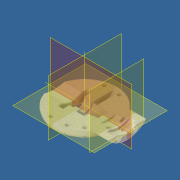
# Autodesk Inventor part: Wrist_B_r1
Saved by Autodesk Inventor 2016 (Build 200138000, 138)
## iProperties
Created: 2016-03-10
Part Number: Wrist_B_r1
Material: ABS-Kunststoff
Document SubType Name: Modeling
Designer: 4ndreas
Density: 1.06 g/cm^3
Appearance: Glatt - weiß
Author: 4ndreas
Autodesk Inventor part; units mm, degrees
sketch "Skizze1" plane through (0, 0, 0) normal (0, 0, 1) x (1, 0, 0)
  circle A0 centre (0, 0) radius 37.5
  line L0 (0, 0) -> (0, 37.5) construction
  dimension "d0" = 75
  constraints: 2 end point, 1 coincident, 1 vertical, 1 vertical alignment, 2 other
extrude "Extrusion1" add sketch "Skizze1" along normal mid plane 58
ref_plane "Arbeitsebene1" through (0, 0, 0) normal (1, 0, 0) x (0, 1, 0)
sketch "Skizze2" plane through (0, 0, 0) normal (1, 0, 0) x (0, 1, 0)
  line L0 (37.5, -29) -> (-37.5, -29) projected
  line L1 (-37.5, -29) -> (-37.5, 29) projected
  line L2 (-37.5, 29) -> (37.5, 29) projected
  line L3 (37.5, 29) -> (37.5, -29) projected
  circle A0 centre (0, 0) radius 29
  constraints: 1 centre point, 1 coincident, 1 tangent
extrude "Extrusion2" add sketch "Skizze2" along normal blind 50 contours A0
ref_plane "Arbeitsebene2" through (0, 0, 0) normal (0, 0, -1) x (-1, 0, 0)
sketch "Skizze3" plane through (50, 0, 0) normal (1, 0, 0) x (0, 0, -1)
  circle A0 centre (0, 0) radius 23.5
  dimension "d7" = 47
  constraints: 1 centre point, 1 coincident
  measures "d7" diameter of A0
extrude "Extrusion3" cut sketch "Skizze3" against normal blind 10
sketch "Skizze4" plane through (40, 0, 0) normal (1, 0, 0) x (0, 0, -1)
  circle A0 centre (0, 0) radius 21
  point P0 (0, 0)
  dimension "d10" = 42
  constraints: 1 centre point, 1 coincident
  measures "d10" diameter of A0
extrude "Extrusion4" cut sketch "Skizze4" against normal blind 12
ref_plane "Arbeitsebene3" through (0, 0, 0) normal (0, -1, 0) x (1, 0, 0)
sketch "Skizze5" plane through (50, 0, 0) normal (1, 0, 0) x (0, 0, -1)
  point P0 (0, 0)
ref_plane "Arbeitsebene4" through (0, 0, 0) normal (1, 0, 0) x (0, 1, 0)
sketch "Skizze6" plane through (0, 0, 0) normal (1, 0, 0) x (0, 1, 0)
  circle A0 centre (20.5107, -9.25) radius 3
  circle A1 centre (0, -18.5) radius 3
  point P0 (0, 0)
  dimension "d13" = 6
  constraints: 2 centre point, 2 coincident, 1 equal radius, 2 other
  measures "d13" diameter of A0
extrude "Extrusion5" cut sketch "Skizze6" along normal mid plane 30
ref_plane "Arbeitsebene5" through (-35, 0, 0) normal (-1, 0, 0) x (0, 1, 0)
ref_plane "Arbeitsebene6" through (-15, 0, 0) normal (1, 0, 0) x (0, -1, 0)
sketch "Skizze8" plane through (-15, 0, 0) normal (1, 0, 0) x (0, -1, 0)
  circle A0 centre (0, 0) radius 5 projected
  circle A1 centre (-25, 0) radius 1.75 projected
  line L0 (14.49, -15.2) -> (27.5875, -2.7143) projected
  arc A2 (27.5875, -2.7143) -> (27.5875, 2.7143) centre (25, 0) ccw projected
  line L1 (27.5875, 2.7143) -> (14.49, 15.2) projected
  arc A3 (14.49, 15.2) -> (-14.49, 15.2) centre (0, 0) ccw projected
  line L2 (-14.49, 15.2) -> (-27.5875, 2.7143) projected
  arc A4 (-27.5875, 2.7143) -> (-27.5875, -2.7143) centre (-25, 0) ccw projected
  line L3 (-27.5875, -2.7143) -> (-14.49, -15.2) projected
  arc A5 (-14.49, -15.2) -> (14.49, -15.2) centre (0, 0) ccw projected
  circle A6 centre (25, 0) radius 1.75 projected
  point P0 (0, 0)
extrude "Extrusion6" cut sketch "Skizze8" against normal through all contours A0 | A1 | A5 L3 A4 L2 A3 L1 A2 L0 | A6
sketch "Skizze9" plane through (28, 0, 0) normal (1, 0, 0) x (0, 0, -1)
  circle A0 centre (0, 0) radius 11
  point P0 (0, 0)
  dimension "d18" = 22
  constraints: 1 centre point, 1 coincident
  measures "d18" diameter of A0
extrude "Extrusion7" cut sketch "Skizze9" against normal blind 7
sketch "Skizze10" plane through (21, 0, 0) normal (1, 0, 0) x (0, 0, -1)
  circle A0 centre (0, 0) radius 6.5
  point P0 (0, 0)
  dimension "d21" = 13
  constraints: 1 centre point, 1 coincident
  measures "d21" diameter of A0
extrude "Extrusion8" cut sketch "Skizze10" against normal through all
ref_plane "Arbeitsebene7" through (50, 0, 0) normal (0, 1, 0) x (-1, 0, 0)
sketch "Skizze11" plane through (50, 0, 0) normal (0, 1, 0) x (-1, 0, 0)
  line L0 (87.5, -29) -> (12.5, -29) projected
  line L1 (0, -29) -> (0, -23.5) projected
  line L2 (0, -23.5) -> (10, -23.5) projected
  line L3 (10, -23.5) -> (10, -21) projected
  line L4 (10, -21) -> (22, -21) projected
  line L5 (22, -21) -> (22, -11) projected
  line L6 (22, -11) -> (29, -11) projected
  line L7 (29, -11) -> (29, -6.5) projected
  line L8 (29, -6.5) -> (65, -6.5) projected
  line L9 (65, 6.5) -> (29, 6.5) projected
  line L10 (29, 6.5) -> (29, 11) projected
  line L11 (29, 11) -> (22, 11) projected
  line L12 (22, 11) -> (22, 21) projected
  line L13 (22, 21) -> (10, 21) projected
  line L14 (10, 21) -> (10, 23.5) projected
  line L15 (10, 23.5) -> (0, 23.5) projected
  line L16 (0, 23.5) -> (0, 29) projected
  line L17 (12.5, 29) -> (87.5, 29) projected
  line L18 (87.5, 29) -> (87.5, 21) projected
  line L19 (87.5, 21) -> (65, 21) projected
  line L20 (65, 21) -> (65, 6.5) projected
  line L21 (65, -15.5) -> (35, -15.5) projected
  line L22 (35, -15.5) -> (35, -21.5) projected
  line L23 (35, -21.5) -> (65, -21.5) projected
  line L24 (65, -21.5) -> (65, -21) projected
  line L25 (65, -21) -> (87.5, -21) projected
  line L26 (87.5, -21) -> (87.5, -29) projected
  line L27 (31, 0) -> (29, 0)
  line L28 (29, 0) -> (29, 9.5)
  line L29 (29, 9.5) -> (31, 9.5)
  line L30 (31, 9.5) -> (31, 0)
  line L31 (87.5, -29) -> (12.5, -29) projected
  line L32 (12.5, -29) -> (0, -29) projected
  line L33 (0, -29) -> (0, -23.5) projected
  line L34 (0, -23.5) -> (10, -23.5) projected
  line L35 (29, -6.5) -> (65, -6.5) projected
  line L36 (65, 6.5) -> (29, 6.5) projected
  line L37 (10, 23.5) -> (0, 23.5) projected
  line L38 (0, 23.5) -> (0, 29) projected
  line L39 (0, 29) -> (12.5, 29) projected
  line L40 (12.5, 29) -> (87.5, 29) projected
  line L41 (87.5, 29) -> (87.5, 21) projected
  line L42 (87.5, 21) -> (65, 21) projected
  line L43 (65, 21) -> (65, 6.5) projected
  line L44 (65, -15.5) -> (35, -15.5) projected
  line L45 (65, -21) -> (87.5, -21) projected
  line L46 (87.5, -21) -> (87.5, -29) projected
  line L47 (-17.7485, 0) -> (106.4912, 0) projected
  line L48 (65, -6.5) -> (65, -15.5) projected
  line L49 (65, -6.5) -> (65, -15.5) projected
  line L50 (35, -15.5) -> (35, -21.5) projected
  line L51 (35, -21.5) -> (65, -21.5) projected
  line L52 (65, -21.5) -> (65, -21) projected
  line L53 (29, 6.5) -> (29, 11) projected
  line L54 (29, 11) -> (22, 11) projected
  line L55 (22, 11) -> (22, 21) projected
  line L56 (22, 21) -> (10, 21) projected
  line L57 (10, 21) -> (10, 23.5) projected
  line L58 (10, -23.5) -> (10, -21) projected
  line L59 (10, -21) -> (22, -21) projected
  line L60 (22, -21) -> (22, -11) projected
  line L61 (22, -11) -> (29, -11) projected
  line L62 (29, -11) -> (29, -6.5) projected
  line L63 (12.5, -29) -> (0, -29) projected
  line L64 (0, 29) -> (12.5, 29) projected
  point P0 (50, 0)
  dimension "d25" = 2
  dimension "d66" = 19
  constraints: 8 end point, 2 collinear, 2 parallel, 1 horizontal, 1 perpendicular
  measures "d25" distance between parallel lines of L30 L28
  measures "d66" diameter of L29 L47
revolve "Umdrehung1" cut sketch "Skizze11" angle 360 about axis through (50, 0, 0) along (-1, 0, 0) contours L30 L27 L28 L9 | L9 L10 L29 L30
ref_plane "Arbeitsebene8" through (50, 0, 0) normal (0, 0, -1) x (-1, 0, 0)
ref_plane "Arbeitsebene9" through (0, 20.5107, -9.25) normal (0, -0.4111111, -0.9115852) x (1, 0, 0)
sketch "Skizze12" plane through (50, 0, 0) normal (0, 1, 0) x (-1, 0, 0)
  line L0 (87.5, 29) -> (87.5, 21) projected
  line L1 (87.5, 21) -> (65, 21) projected
  line L2 (65, 21) -> (65, 6.5) projected
  line L3 (65, 6.5) -> (31, 6.5) projected
  line L4 (31, 6.5) -> (31, 9.5) projected
  line L5 (31, 9.5) -> (29, 9.5) projected
  line L6 (29, 9.5) -> (29, 11) projected
  line L7 (29, 11) -> (22, 11) projected
  line L8 (22, 11) -> (22, 21) projected
  line L9 (22, 21) -> (10, 21) projected
  line L10 (10, 21) -> (10, 23.5) projected
  line L11 (10, 23.5) -> (0, 23.5) projected
  line L12 (0, 23.5) -> (0, 29) projected
  line L13 (12.5, 29) -> (87.5, 29) projected
  line L14 (87.5, -29) -> (12.5, -29) projected
  line L15 (0, -29) -> (0, -23.5) projected
  line L16 (0, -23.5) -> (10, -23.5) projected
  line L17 (10, -23.5) -> (10, -21) projected
  line L18 (10, -21) -> (22, -21) projected
  line L19 (22, -21) -> (22, -11) projected
  line L20 (22, -11) -> (29, -11) projected
  line L21 (29, -11) -> (29, -9.5) projected
  line L22 (29, -9.5) -> (31, -9.5) projected
  line L23 (31, -9.5) -> (31, -6.5) projected
  line L24 (31, -6.5) -> (65, -6.5) projected
  line L25 (65, -6.5) -> (65, -15.5) projected
  line L26 (65, -15.5) -> (35, -15.5) projected
  line L27 (35, -15.5) -> (35, -21.5) projected
  line L28 (35, -21.5) -> (65, -21.5) projected
  line L29 (65, -21.5) -> (65, -21) projected
  line L30 (65, -21) -> (87.5, -21) projected
  line L31 (87.5, -21) -> (87.5, -29) projected
  line L32 (105, -18.5) -> (-17.5, -18.5) projected
  line L33 (54, -18.5) -> (34, -18.5)
  line L34 (34, -18.5) -> (34, -25)
  line L35 (34, -25) -> (54, -25)
  line L36 (54, -25) -> (54, -18.5)
  line L37 (65, -20.9257) -> (65, -15.5) projected
  line L38 (49, -25) -> (39, -25)
  line L39 (39, -25) -> (39, -27.5)
  line L40 (39, -27.5) -> (49, -27.5)
  line L41 (49, -27.5) -> (49, -25)
  line L42 (54, -27.5) -> (59, -27.5)
  line L43 (59, -27.5) -> (59, -18.5)
  line L44 (59, -18.5) -> (54, -18.5)
  line L45 (54, -18.5) -> (54, -27.5)
  line L46 (59, -18.5) -> (65, -18.5)
  line L47 (65, -18.5) -> (65, -35)
  line L48 (65, -35) -> (59, -35)
  line L49 (59, -35) -> (59, -18.5)
  line L50 (12.5, -29) -> (0, -29) projected
  line L51 (0, 29) -> (12.5, 29) projected
  line L52 (54, -27.5) -> (59, -27.5)
  line L53 (59, -27.5) -> (59, -18.5)
  line L54 (59, -18.5) -> (54, -18.5)
  line L55 (54, -18.5) -> (54, -27.5)
  line L56 (34, -18.5) -> (39, -18.5)
  line L57 (39, -18.5) -> (39, -25)
  line L58 (39, -25) -> (34, -25)
  line L59 (34, -25) -> (34, -18.5)
  line L60 (34, -18.5) -> (29, -18.5)
  line L61 (29, -18.5) -> (29, -24)
  line L62 (29, -24) -> (34, -24)
  line L63 (34, -24) -> (34, -18.5)
  line L64 (54, -18.5) -> (48, -18.5)
  line L65 (48, -18.5) -> (48, -28)
  line L66 (48, -28) -> (54, -28)
  line L67 (54, -28) -> (54, -18.5)
  point P0 (50, 0)
  dimension "d30" = 20
  dimension "d31" = 11
  dimension "d57" = 5
  dimension "d58" = 5
  dimension "d59" = 18
  dimension "d60" = 33
  dimension "d61" = 5
  dimension "d62" = 6
  dimension "d136" = 13
  dimension "d142" = 13
  dimension "d143" = 5
  dimension "d144" = 18
  dimension "d145" = 11
  dimension "d146" = 19
  dimension "d147" = 6
  constraints: 64 end point, 16 parallel, 8 horizontal, 8 perpendicular, 5 point on line, 2 collinear
  measures "d30" distance between parallel lines of L34 L36
  measures "d31" distance between parallel lines of L36 L37
  measures "d57" distance between parallel lines of L36 L41
  measures "d58" distance between parallel lines of L39 L34
  measures "d59" diameter of L42 L32
  measures "d60" diameter of L48 L32
  measures "d61" distance between parallel lines of L43 L45
  measures "d62" distance between parallel lines of L47 L49
  measures "d136" diameter of L35 L32
  measures "d142" diameter of L58 L32
  measures "d143" distance between parallel lines of L34 L61
  measures "d144" diameter of L40 L32
  measures "d145" diameter of L62 L32
  measures "d146" diameter of L66 L32
  measures "d147" distance between parallel lines of L36 L65
revolve "Umdrehung2" cut sketch "Skizze12" angle 360 about axis through (0, 0, -18.5) along (1, 0, 0) contours L47 L48 L49 L14 | L14 L49 L43 L28 L47 | L28 L43 L32 L37 L47 L29 | L42 L45 L36 L28 L43 | L28 L36 L32 L43 | L36 L35 L65 L28 | L28 L65 L32 L36 | L65 L35 L57 L28 | L28 L57 L32 L65 | L41 L40 L65 L35 | L57 L35 L34 L32 L27 L28 | L28 L27 L32 L57 | L65 L40 L39 L35 | L34 L62 L61 L32
sketch "Skizze13" plane through (0, 20.5107, -9.25) normal (0, -0.4111111, -0.9115852) x (1, 0, 0)
  line L0 (-15, -1.2682) -> (-15, 0.9858) projected
  line L1 (-15, 0.9858) -> (-15, -1.2682) projected
  line L2 (15, -3) -> (15, 3) projected
  line L3 (-31.2952, -0.1645) -> (-15, -0.1645) projected
  line L4 (-15, -0.1645) -> (-15, -3) projected
  line L5 (-15, -3) -> (15, -3) projected
  line L6 (15, 3) -> (-15, 3) projected
  line L7 (-15, 3) -> (-15, 16) projected
  line L8 (-15, 16) -> (19, 16) projected
  line L9 (19, 16) -> (19, 13) projected
  line L10 (19, 13) -> (21, 13) projected
  line L11 (21, 13) -> (21, 11.5) projected
  line L12 (21, 11.5) -> (28, 11.5) projected
  line L13 (28, 11.5) -> (28, 1.5) projected
  line L14 (28, 1.5) -> (40, 1.5) projected
  line L15 (40, 1.5) -> (40, -1) projected
  line L16 (40, -1) -> (50, -1) projected
  line L17 (50, -1) -> (50, -6.5) projected
  line L18 (50, -6.5) -> (26.5968, -6.5) projected
  line L19 (26.5968, 51.5) -> (50, 51.5) projected
  line L20 (50, 51.5) -> (50, 46) projected
  line L21 (50, 46) -> (40, 46) projected
  line L22 (40, 46) -> (40, 43.5) projected
  line L23 (40, 43.5) -> (28, 43.5) projected
  line L24 (28, 43.5) -> (28, 33.5) projected
  line L25 (28, 33.5) -> (21, 33.5) projected
  line L26 (21, 33.5) -> (21, 32) projected
  line L27 (21, 32) -> (19, 32) projected
  line L28 (19, 32) -> (19, 29) projected
  line L29 (19, 29) -> (-15, 29) projected
  line L30 (-15, 29) -> (-15, 45.1645) projected
  line L31 (-15, 45.1645) -> (-31.2952, 45.1645) projected
  line L32 (-55, 0) -> (67.5, 0) projected
  line L33 (24, 0) -> (-4, 0)
  line L34 (-4, 0) -> (-4, 6.5)
  line L35 (-4, 6.5) -> (14, 6.5)
  line L36 (24, 6.5) -> (24, 0)
  line L37 (-15, 3) -> (-15, -1.2682) projected
  line L38 (28, 0) -> (24, 0)
  line L39 (24, 0) -> (24, 8)
  line L40 (24, 8) -> (28, 8)
  line L41 (28, 8) -> (28, 0)
  line L42 (34, 0) -> (28, 0)
  line L43 (28, 0) -> (28, 9)
  line L44 (28, 9) -> (34, 9)
  line L45 (34, 9) -> (34, 0)
  line L46 (1, 0) -> (7, 0)
  line L47 (7, 0) -> (7, 16)
  line L48 (7, 16) -> (1, 16)
  line L49 (1, 16) -> (1, 0)
  ellipse E0 centre (0, 22.5) end of major axis (0, 63.6371) minor radius 37.5 (-31.2952, -0.1645) -> (26.5968, -6.5) ccw projected
  ellipse E1 centre (0, 22.5) end of major axis (0, 63.6371) minor radius 37.5 (26.5968, 51.5) -> (-31.2952, 45.1645) ccw projected
  line L50 (15, -3) -> (15, 3) projected
  line L51 (14, 6.5) -> (19, 6.5)
  line L52 (19, 6.5) -> (19, 5.5)
  line L53 (19, 5.5) -> (14, 5.5)
  line L54 (14, 5.5) -> (14, 6.5)
  line L55 (14, 6.5) -> (19, 6.5)
  line L56 (19, 6.5) -> (24, 6.5)
  dimension "d35" = 28
  dimension "d36" = 11
  dimension "d39" = 9
  dimension "d40" = 4
  dimension "d41" = 6
  dimension "d63" = 5
  dimension "d64" = 6
  dimension "d65" = 32
  dimension "d137" = 13
  dimension "d138" = 16
  dimension "d139" = 5
  dimension "d140" = 1
  dimension "d141" = 5
  constraints: 44 end point, 12 parallel, 5 horizontal, 5 perpendicular, 5 point on line, 1 collinear, 2 other
  measures "d35" distance between parallel lines of L34 L36
  measures "d36" distance between parallel lines of L34 L37
  measures "d39" distance between parallel lines of L42 L44
  measures "d40" distance between parallel lines of L41 L39
  measures "d41" distance between parallel lines of L43 L45
  measures "d63" distance between parallel lines of L34 L49
  measures "d64" distance between parallel lines of L47 L49
  measures "d65" diameter of L48 L32
  measures "d137" diameter of L35 L32
  measures "d138" diameter of L40 L32
  measures "d139" distance between parallel lines of L52 L36
  measures "d140" distance between parallel lines of L55 L53
  measures "d141" distance between parallel lines of L54 L52
revolve "Umdrehung3" cut sketch "Skizze13" angle 360 about axis through (0, 20.5107, -9.25) along (1, 0, 0) contours L34 L6 L49 L32 | L32 L47 L6 L2 | L2 L6 L47 L35 L54 L53 L52 L56 L36 L32 | L49 L6 L47 L32 | L34 L35 L49 L6 | L36 L39 L40 L13 L41 L32 | L49 L35 L47 L6 | L41 L14 L45 L32 | L8 L47 L35 L49 | L13 L44 L45 L14
sketch "Skizze14" plane through (50, 0, 0) normal (0, 1, 0) x (-1, 0, 0)
  point P0 (50, 0)
sketch "Skizze15" plane through (0, 0, 29) normal (0, 0, 1) x (1, 0, 0)
  circle A0 centre (0, 0) radius 11.5
  dimension "d42" = 23
  constraints: 1 centre point, 1 coincident
  measures "d42" diameter of A0
extrude "Extrusion9" cut sketch "Skizze15" against normal blind 29
sketch "Skizze16" plane through (0, 0, 29) normal (0, 0, 1) x (1, 0, 0)
  line L0 (-5.9316, 14.3201) -> (5.9316, 14.3201) construction
  line L1 (5.9316, 14.3201) -> (14.3201, 5.9316) construction
  line L2 (14.3201, 5.9316) -> (14.3201, -5.9316) construction
  line L3 (14.3201, -5.9316) -> (5.9316, -14.3201) construction
  line L4 (5.9316, -14.3201) -> (-5.9316, -14.3201) construction
  line L5 (-5.9316, -14.3201) -> (-14.3201, -5.9316) construction
  line L6 (-14.3201, -5.9316) -> (-14.3201, 5.9316) construction
  line L7 (-14.3201, 5.9316) -> (-5.9316, 14.3201) construction
  circle A0 centre (0, 0) radius 15.5 construction
  line L8 (-55.0017, 0) -> (67.5003, 0) projected
  line L9 (0, 52.5) -> (0, -52.5) projected
  dimension "d45" = 31
  constraints: 16 end point, 2 coincident, 1 midpoint, 1 parallel, 1 point on line, 20 other
hole "Bohrung1" at (-5.9316, 14.3201, 29) at (14.3201, 5.9316, 29) at (5.9316, 14.3201, 29) at (14.3201, -5.9316, 29) at (5.9316, -14.3201, 29) at (-5.9316, -14.3201, 29) at (-14.3201, -5.9316, 29) at (-14.3201, 5.9316, 29) direction (0, 0, -1) diameter 3 depth 2
sketch "Skizze17" plane through (50, 0, 0) normal (1, 0, 0) x (0, 0, -1)
  circle A0 centre (0, 0) radius 23.5 projected
  circle A1 centre (0, 0) radius 21.5
  dimension "d53" = 43
  constraints: 1 centre point, 1 coincident
  measures "d53" diameter of A1
extrude "Extrusion10" add sketch "Skizze17" against normal blind 3
ref_plane "Arbeitsebene10" through (0, 20.5107, -9.25) normal (0, 0, 1) x (1, 0, 0)
ref_plane "Arbeitsebene11" through (0, 0, -18.5) normal (0, 0, 1) x (1, 0, 0)
sketch "Skizze18" plane through (-15, 0, 0) normal (1, 0, 0) x (0, 0, -1)
  arc A0 (11.4276, 18.4472) -> (7.293, 22.7845) centre (9.25, 20.5107) ccw projected
  circle A1 centre (9.25, 20.5107) radius 3
  line L0 (7.293, 22.7845) -> (11.4276, 18.4472) projected
  point P0 (0, 0)
  constraints: 1 centre point, 1 coincident, 1 concentric
extrude "Extrusion11" add sketch "Skizze18" along normal blind 5
fillet "Rundung2" radius 8 2 edges at (-12, -5.7486, -3.0338) (-12, 5.7486, -3.0338)
sketch "Skizze20" plane through (50, 0, 0) normal (1, 0, 0) x (0, 0, -1)
  circle A0 centre (0, 0) radius 21.5 projected
  circle A1 centre (0, 0) radius 29 projected
  line L0 (-20.5061, 20.5061) -> (-29, 12.0122)
  line L1 (-29, 12.0122) -> (-29, -12.0122)
  line L2 (-29, -12.0122) -> (-20.5061, -20.5061)
  line L3 (20.5061, -20.5061) -> (29, -12.0122)
  line L4 (29, -12.0122) -> (29, 12.0122)
  line L5 (29, 12.0122) -> (20.5061, 20.5061)
  circle A2 centre (0, 0) radius 29 projected
  dimension "d74" = 135
  constraints: 12 end point, 5 tangent, 4 equal length, 4 point on circle, 1 parallel, 1 vertical
  measures "d74" angle of L4 L5
extrude "Extrusion13" add sketch "Skizze20" against normal up to surface contours L4 L3 A1 | A1 L5 L4 | A1 L1 L0 | L2 L1 A1 round surface about axis through (0, 0, 0) along (0, 0, 1) radius 37.5 far side no
sketch "Skizze21" plane through (50, 0, 0) normal (1, 0, 0) x (0, 0, -1)
  circle A0 centre (0, 0) radius 21.5 projected
  arc A1 (20.5061, 20.5061) -> (-20.5061, 20.5061) centre (0, 0) ccw projected
  line L0 (-20.5061, 20.5061) -> (-29, 12.0122) projected
  line L1 (-29, 12.0122) -> (-29, -12.0122) projected
  line L2 (-29, -12.0122) -> (-20.5061, -20.5061) projected
  arc A2 (-20.5061, -20.5061) -> (20.5061, -20.5061) centre (0, 0) ccw projected
  line L3 (20.5061, -20.5061) -> (29, -12.0122) projected
  line L4 (29, -12.0122) -> (29, 12.0122) projected
  line L5 (29, 12.0122) -> (20.5061, 20.5061) projected
  circle A3 centre (0, 0) radius 29
  constraints: 1 centre point, 1 coincident, 1 concentric
extrude "Extrusion14" cut sketch "Skizze21" against normal blind 6.5 contours L5 L4 A3 | A3 L1 L0 | L4 L3 A3 | A3 L2 L1
ref_plane "Arbeitsebene12" through (43.5, 0, 0) normal (1, 0, 0) x (0, 0, -1)
ref_plane "Arbeitsebene13" through (-9, -12.7279, -29) normal (-1, 0, 0) x (0, 0, 1)
sketch "Skizze22" plane through (0, 0, 29) normal (0, 0, 1) x (1, 0, 0)
  point P0 (0, 0)
sketch "Skizze23" plane through (0, 0, 29) normal (0, 0, 1) x (1, 0, 0)
  circle A0 centre (0, 0) radius 32.5 construction
  line L0 (-9.5, -6.4938) -> (-9.5, -9.6574) construction
  line L1 (1, 8.8391) -> (1, 4.5815) construction
  line L2 (-15, -14.49) -> (-15, 14.49) construction
  line L3 (-15, -14.49) -> (-15, -27.5875) construction
  line L4 (-15, -28.75) -> (-24.0767, -28.75) construction
  line L5 (-15, -27.5875) -> (-25.4004, -27.5875) construction
  line L6 (-15, -14.49) -> (-34.5874, -14.49) construction
  line L7 (-15, 28.75) -> (-24.0767, 28.75) construction
  line L8 (-15, 27.5875) -> (-25.4004, 27.5875) construction
  line L9 (-15, 27.5875) -> (-15, 14.49) construction
  line L10 (-10, 23.5107) -> (-4, 23.5107) construction
  line L11 (-10, 17.5107) -> (-4, 17.5107) construction
  line L12 (-10, 23.5107) -> (-10, 17.5107) construction
  circle A1 centre (0, 0) radius 11.5 construction
  circle A2 centre (-14.3201, 5.9316) radius 1.5 construction
  circle A3 centre (-5.9316, -14.3201) radius 1.5 construction
  circle A4 centre (14.3201, -5.9316) radius 1.5 construction
  circle A5 centre (14.3201, 5.9316) radius 1.5 construction
  circle A6 centre (-5.9316, 14.3201) radius 1.5 construction
  circle A7 centre (5.9316, 14.3201) radius 1.5 construction
  circle A8 centre (5.9316, -14.3201) radius 1.5 construction
  circle A9 centre (-14.3201, -5.9316) radius 1.5 construction
  line L13 (43.5, -12.0122) -> (43.5, 0) construction
  line L14 (43.5, 0) -> (43.5, 12.0122) construction
  line L15 (43.5, 12.0122) -> (35.524, 12.0122) construction
  arc A10 (35.524, 12.0122) -> (35.524, -12.0122) centre (0, 0) ccw construction
  line L16 (43.5, -12.0122) -> (35.524, -12.0122) construction
  line L17 (28, 28.5347) -> (28, 20.9984) construction
  line L18 (29.7977, 22.7673) -> (34, 22.7673) construction
  line L19 (34, 28.5347) -> (34, 20.9984) construction
  line L20 (23.775, -29) -> (50, -29) construction
  line L21 (0, 0) -> (10.0431, 30.9093) construction
  line L22 (0, 0) -> (-8.4116, 31.3926) construction
  line L23 (-8.4116, -31.3926) -> (0, 0) construction
  line L24 (0, 0) -> (10.0431, -30.9093) construction
  line L25 (0, 0) -> (0, -32.5) construction
  line L26 (0, 0) -> (22.981, -22.981) construction
  line L27 (1, 36.5107) -> (1, 8.8391) construction
  point P0 (1, 4.5815)
  point P1 (-5, 13.0107)
  point P2 (7, 14.0107)
  point P3 (1, 11.4564)
  point P4 (1, 5.9253)
  dimension "d85" = 5
  dimension "d121" = 15
  dimension "d122" = 18
  dimension "d123" = 15
  dimension "d124" = 18
  dimension "d125" = 45
  constraints: 14 end point, 6 point on circle, 1 centre point, 1 coincident, 1 vertical, 2 other
  measures "d85" radial gap between concentric circles of A10 A0
  measures "d121" angle of L23 L25
  measures "d122" angle of L24 L25
  measures "d123" angle of L27 L22
  measures "d124" angle of L27 L21
  measures "d125" angle of L26 L25
hole "Bohrung2" at (-8.4116, -31.3926, 29) at (-8.4116, 31.3926, 29) at (10.0431, 30.9093, 29) at (10.0431, -30.9093, 29) at (22.981, -22.981, 29) direction (0, 0, -1) diameter 4 end through all counterbore diameter 7 counterbore depth 4
sketch "Skizze24" plane through (50, 0, 0) normal (0, 0, -1) x (-1, 0, 0)
  circle A0 centre (39.9569, 30.9093) radius 2 projected
  circle A1 centre (58.4116, -31.3926) radius 2 projected
  circle A2 centre (58.4116, 31.3926) radius 2 projected
  circle A3 centre (39.9569, -30.9093) radius 2 projected
  line L0 (31, -9.5) -> (31, -6.5) projected
  line L1 (31, -6.5) -> (40.5132, -6.5) projected
  line L2 (29, -9.5) -> (31, -9.5) projected
  line L3 (29, -11) -> (29, -9.5) projected
  line L4 (22, -11) -> (29, -11) projected
  line L5 (22, -21) -> (22, -11) projected
  line L6 (10, -21) -> (22, -21) projected
  line L7 (10, -23.5) -> (10, -21) projected
  line L8 (3, -23.5) -> (10, -23.5) projected
  line L9 (3, -21.5) -> (3, -23.5) projected
  line L10 (0, -21.5) -> (3, -21.5) projected
  line L11 (0, -29) -> (0, -21.5) projected
  line L12 (26.225, -29) -> (0, -29) projected
  arc A4 (26.225, -29) -> (74.0767, -28.75) centre (50, 0) ccw projected
  line L13 (65, -28.75) -> (74.0767, -28.75) projected
  line L14 (65, -6.5472) -> (65, -28.75) projected
  line L15 (31, 6.5) -> (31, 9.5) projected
  line L16 (31, 9.5) -> (29, 9.5) projected
  line L17 (29, 9.5) -> (29, 11) projected
  line L18 (29, 11) -> (22, 11) projected
  line L19 (22, 11) -> (22, 21) projected
  line L20 (22, 21) -> (10, 21) projected
  line L21 (10, 21) -> (10, 23.5) projected
  line L22 (10, 23.5) -> (3, 23.5) projected
  line L23 (3, 23.5) -> (3, 21.5) projected
  line L24 (3, 21.5) -> (0, 21.5) projected
  line L25 (0, 21.5) -> (0, 29) projected
  line L26 (0, 29) -> (26.225, 29) projected
  arc A5 (74.0767, 28.75) -> (26.225, 29) centre (50, 0) ccw projected
  line L27 (74.0767, 28.75) -> (65, 28.75) projected
  line L28 (65, 28.75) -> (65, 6.5472) projected
  line L29 (59, 6.5) -> (40.5132, 6.5) projected
  line L30 (40.5132, 6.5) -> (31, 6.5) projected
  line L31 (49, 33.5658) -> (43, 33.5658) projected
  line L32 (43, 33.5658) -> (43, 9.1241) projected
  line L33 (43, 7.4555) -> (49, 7.4555) projected
  line L34 (43, 9.1241) -> (43, 7.4555) projected
  line L35 (39.9569, 34.9508) -> (43.4569, 32.9301)
  line L36 (43.4569, 32.9301) -> (43.4569, 28.8886)
  line L37 (43.4569, 28.8886) -> (39.9569, 26.8679)
  line L38 (39.9569, 26.8679) -> (36.4569, 28.8886)
  line L39 (36.4569, 28.8886) -> (36.4569, 32.9301)
  line L40 (36.4569, 32.9301) -> (39.9569, 34.9508)
  line L41 (58.4116, 27.3511) -> (54.9116, 29.3719)
  line L42 (54.9116, 29.3719) -> (54.9116, 33.4133)
  line L43 (54.9116, 33.4133) -> (58.4116, 35.434)
  line L44 (58.4116, 35.434) -> (61.9116, 33.4133)
  line L45 (61.9116, 33.4133) -> (61.9116, 29.3719)
  line L46 (61.9116, 29.3719) -> (58.4116, 27.3511)
  line L47 (30.519, -25.0017) -> (27.019, -27.0224)
  line L48 (27.019, -27.0224) -> (23.519, -25.0017)
  line L49 (23.519, -25.0017) -> (23.519, -20.9602)
  line L50 (23.519, -20.9602) -> (27.019, -18.9395)
  line L51 (27.019, -18.9395) -> (30.519, -20.9602)
  line L52 (30.519, -20.9602) -> (30.519, -25.0017)
  line L53 (39.9569, -26.8679) -> (43.4569, -28.8886)
  line L54 (43.4569, -28.8886) -> (43.4569, -32.9301)
  line L55 (43.4569, -32.9301) -> (39.9569, -34.9508)
  line L56 (39.9569, -34.9508) -> (36.4569, -32.9301)
  line L57 (36.4569, -32.9301) -> (36.4569, -28.8886)
  line L58 (36.4569, -28.8886) -> (39.9569, -26.8679)
  line L59 (61.9116, -29.3719) -> (61.9116, -33.4133)
  line L60 (61.9116, -33.4133) -> (58.4116, -35.434)
  line L61 (58.4116, -35.434) -> (54.9116, -33.4133)
  line L62 (54.9116, -33.4133) -> (54.9116, -29.3719)
  line L63 (54.9116, -29.3719) -> (58.4116, -27.3511)
  line L64 (58.4116, -27.3511) -> (61.9116, -29.3719)
  circle A6 centre (27.019, -22.981) radius 2 projected
  line L65 (49, 11.4564) -> (49, 33.5658) projected
  line L66 (49, 7.4555) -> (49, 11.4564) projected
  arc A7 (40.5132, -6.5) -> (59.4543, -6.5472) centre (50, 0) ccw projected
  line L67 (59, -6.5472) -> (59.4543, -6.5472) projected
  line L68 (59, -6.5) -> (59, -6.5472) projected
  line L69 (40.5132, -6.5) -> (59, -6.5) projected
  line L70 (59.4543, -6.5472) -> (65, -6.5472) projected
  line L71 (65, 6.5472) -> (59.4543, 6.5472) projected
  line L72 (59.4543, 6.5472) -> (59, 6.5472) projected
  line L73 (59, 6.5472) -> (59, 6.5) projected
  arc A8 (59.4543, 6.5472) -> (49, 11.4564) centre (50, 0) ccw projected
  arc A9 (43, 9.1241) -> (40.5132, 6.5) centre (50, 0) ccw projected
  point P0 (50, 0)
  point P1 (50, 11.5)
  point P2 (50, 7.4555)
  point P3 (27.019, -22.981)
  point P4 (27.019, -22.981)
  dimension "d102" = 7
  constraints: 60 end point, 5 coincident, 4 equal length, 4 parallel, 65 other
  measures "d102" distance between parallel lines of L45 L42
extrude "Extrusion15" cut sketch "Skizze24" along normal mid plane 20 contours A0 | A1 | A2 | A3 | L37 L38 L39 L40 L35 L32 | L32 L35 L36 L37 | L41 L42 L43 L44 L45 L46 | L47 L48 L49 L50 L51 L52 | L53 L54 L55 L56 L57 L58 | L59 L60 L61 L62 L63 L64 | A6
sketch "Skizze25" plane through (-15, 0, 0) normal (-1, 0, 0) x (0, 0, 1)
  arc A0 (0.5785, -6.4742) -> (0.5785, 6.4742) centre (0, 0) ccw projected
  line L0 (-2.7143, -27.5875) -> (-13.9059, -15.8475) projected
  arc A1 (-2.7143, -27.5875) -> (2.7143, -27.5875) centre (0, -25) ccw projected
  line L1 (15.2, -14.49) -> (2.7143, -27.5875) projected
  arc A2 (15.2, -14.49) -> (15.2, 14.49) centre (0, 0) ccw projected
  line L2 (2.7143, 27.5875) -> (15.2, 14.49) projected
  arc A3 (2.7143, 27.5875) -> (-2.7143, 27.5875) centre (0, 25) ccw projected
  line L3 (-13.9059, 15.8475) -> (-2.7143, 27.5875) projected
  arc A4 (-5.1717, 9.7266) -> (0.5785, 6.4742) centre (1.2905, 14.4425) ccw projected
  arc A5 (0.5785, -6.4742) -> (-5.1717, -9.7266) centre (1.2905, -14.4425) ccw projected
  arc A6 (-13.9059, -15.8475) -> (-5.1717, -9.7266) centre (-18.5, 0) ccw projected
  arc A7 (-5.1717, 9.7266) -> (-13.9059, 15.8475) centre (-18.5, 0) ccw projected
  point P0 (0, 0)
hole "Bohrung4" at (-15, -25, 0) at (-15, 25, 0) direction (1, 0, 0) diameter 2.5 depth 10
fillet "Rundung3" radius 8 2 edges at (-37.5, 0, -29) (-37.5, 0, 29)
mirror "Spiegeln2" about plane through (50, 0, 0) normal (0, 0, -1) of "Bohrung2"
mirror "Spiegeln3" about plane through (50, 0, 0) normal (0, 0, -1) of "Bohrung1"
sketch "Skizze31" plane through (50, 0, 0) normal (1, 0, 0) x (0, 0, -1)
  circle A0 centre (0, 0) radius 29 projected
  circle A1 centre (0, 0) radius 21 projected
  circle A2 centre (0, 0) radius 23.5 projected
  line L0 (-9.5671, -23.097) -> (-23.097, -9.5671) construction
  line L1 (-23.097, -9.5671) -> (-23.097, 9.5671) construction
  line L2 (-23.097, 9.5671) -> (-9.5671, 23.097) construction
  line L3 (-9.5671, 23.097) -> (9.5671, 23.097) construction
  line L4 (9.5671, 23.097) -> (23.097, 9.5671) construction
  line L5 (23.097, 9.5671) -> (23.097, -9.5671) construction
  line L6 (23.097, -9.5671) -> (9.5671, -23.097) construction
  line L7 (9.5671, -23.097) -> (-9.5671, -23.097) construction
  line L8 (-40.6, 0) -> (40.6, 0) construction
  circle A3 centre (9.5671, -23.097) radius 4 construction
  circle A4 centre (9.5671, -23.097) radius 1.5 construction
  circle A5 centre (0, 0) radius 25
  line L9 (9.25, -52.5) -> (9.25, 52.5) projected
  line L10 (0, 52.5) -> (0, -52.5) projected
  circle A6 centre (4.625, -24.5685) radius 4.625 construction
  line L11 (18.5, -52.5) -> (18.5, 52.5) construction
  circle A7 centre (13.875, -20.7963) radius 4.625 construction
  circle A8 centre (13.875, 20.7963) radius 4.625 construction
  circle A9 centre (4.625, 24.5685) radius 4.625 construction
  point P0 (0, 0)
  dimension "d126" = 3
  constraints: 16 end point, 10 tangent, 7 centre point, 5 point on circle, 4 coincident, 1 parallel, 17 other
  measures "d126" diameter of A4
hole "Bohrung5" at (50, -23.097, 9.5671) at (50, -9.5671, 23.097) at (50, 9.5671, 23.097) at (50, 23.097, 9.5671) at (50, -9.5671, -23.097) at (50, 9.5671, -23.097) at (50, -24.5685, -4.625) at (50, -20.7963, -13.875) at (50, 20.7963, -13.875) at (50, 24.5685, -4.625) direction (-1, 0, 0) diameter 2.5 depth 20 countersink diameter 6 countersink angle 90
thicken "Verdickung1" operation cut thickness 1 both sides no extend neighbours no toward (0, -0.69, -0.7238094) faces at (-18.4668, -23.6742, -6.4448) (-29.3074, 7.939, -19.4415) (-21.7115, -27.8077, 2.4858) (-19.5021, -22.1474, 7.9002) (-29.3074, 7.939, 19.4415) (-20.0591, 21.4463, 8.5686) (-21.7115, 27.8077, -2.4858) (-19.5021, 22.5999, -7.4689)
sketch "Skizze32" plane through (0, 0, -29) normal (0, 0, -1) x (-1, 0, 0)
  circle A0 centre (0, 0) radius 11.5 projected
  line L0 (9.4543, -6.5472) -> (9, -6.5472) projected
  arc A1 (-9.4868, -6.5) -> (9.4543, -6.5472) centre (0, 0) ccw projected
  line L1 (9, -6.5) -> (-9.4868, -6.5) projected
  line L2 (9, -6.5472) -> (9, -6.5) projected
  line L3 (-1, 11.4564) -> (-1, 7.4555) projected
  line L4 (-1, 5.9253) -> (-1, 7.4555) projected
  line L5 (-1, 4.5815) -> (-1, 5.9253) projected
  line L6 (-1, 8.8391) -> (-1, 4.5815) projected
  line L7 (-1, 11.4564) -> (-1, 8.8391) projected
  line L8 (-1, 27.0107) -> (-1, 14.0107) projected
  line L9 (-1, -6.5) -> (-1, 6.5) projected
  line L10 (0, -52.5) -> (0, 52.5) projected
  line L11 (-1, -6.5) -> (4, -6.5) projected
  line L12 (-11, -9) -> (-1, -9) projected
  line L13 (-16, -6.5) -> (-11, -6.5) projected
  line L14 (-21, -5.5) -> (-16, -5.5) projected
  line L15 (-1, -6.9) -> (-11, -6.9)
  line L16 (-11, -6.9) -> (-11, -11.5)
  line L17 (-11, -11.5) -> (-1, -11.5)
  line L18 (-1, -11.5) -> (-1, -6.9)
  dimension "d150" = 0.4
  constraints: 8 end point, 2 parallel, 2 point on line, 1 horizontal, 1 perpendicular, 1 tangent
  measures "d150" distance between parallel lines of L1 L15
extrude "Extrusion17" cut sketch "Skizze32" against normal up to surface (29 mm away) contours L15 L18 L12 A0 | A0 L12 L16 L15 | L12 L18 A0 | A0 L18 L17 L16 L12
ref_plane "Arbeitsebene14" through (38, 0, 0) normal (1, 0, 0) x (0, 0, -1)
sketch "Skizze33" plane through (38, 0, 0) normal (1, 0, 0) x (0, 0, -1)
  circle A0 centre (13.875, 20.7963) radius 1.25 projected
  circle A1 centre (4.625, -24.5685) radius 1.25 projected
  circle A2 centre (23.097, -9.5671) radius 1.25 projected
  circle A3 centre (-23.097, 9.5671) radius 1.25 projected
  circle A4 centre (-9.5671, -23.097) radius 1.25 projected
  circle A5 centre (-23.097, -9.5671) radius 1.25 projected
  circle A6 centre (-9.5671, 23.097) radius 1.25 projected
  circle A7 centre (23.097, 9.5671) radius 1.25 projected
  circle A8 centre (13.875, -20.7963) radius 1.25 projected
  circle A9 centre (4.625, 24.5685) radius 1.25 projected
  line L0 (-20.5061, -20.5061) -> (-29, -12.0122) projected
  line L1 (-29, -12.0122) -> (-29, 12.0122) projected
  line L2 (-29, 12.0122) -> (-20.5061, 20.5061) projected
  arc A10 (20.5061, 20.5061) -> (-20.5061, 20.5061) centre (0, 0) ccw projected
  line L3 (20.5061, 20.5061) -> (29, 12.0122) projected
  line L4 (29, 12.0122) -> (29, -12.0122) projected
  line L5 (29, -12.0122) -> (20.5061, -20.5061) projected
  arc A11 (-20.5061, -20.5061) -> (20.5061, -20.5061) centre (0, 0) ccw projected
  circle A12 centre (0, 0) radius 21 projected
  line L6 (12.4686, -23.6432) -> (10.7062, -21.0018)
  line L7 (10.7062, -21.0018) -> (12.1126, -18.1548)
  line L8 (12.1126, -18.1548) -> (15.2814, -17.9493)
  line L9 (15.2814, -17.9493) -> (17.0438, -20.5907)
  line L10 (17.0438, -20.5907) -> (15.6374, -23.4377)
  line L11 (15.6374, -23.4377) -> (12.4686, -23.6432)
  line L12 (0, 0) -> (13.875, -20.7963) construction
  line L13 (10.7062, -21.0018) -> (15.2814, -17.9493)
  line L14 (15.2814, -17.9493) -> (7.3128, -6.0056)
  line L15 (7.3128, -6.0056) -> (2.7376, -9.0581)
  line L16 (2.7376, -9.0581) -> (10.7062, -21.0018)
  line L17 (0, 0) -> (23.097, -9.5671) construction
  line L18 (0, 0) -> (4.625, -24.5685) construction
  line L19 (0, 0) -> (-9.5671, -23.097) construction
  line L20 (0, 0) -> (-23.097, -9.5671) construction
  line L21 (23.5115, -12.7153) -> (20.5778, -11.5002)
  line L22 (20.5778, -11.5002) -> (20.1633, -8.3519)
  line L23 (20.1633, -8.3519) -> (22.6825, -6.4188)
  line L24 (22.6825, -6.4188) -> (25.6162, -7.634)
  line L25 (25.6162, -7.634) -> (26.0307, -10.7823)
  line L26 (26.0307, -10.7823) -> (23.5115, -12.7153)
  line L27 (1.6287, -23.5169) -> (4.0375, -21.4478)
  line L28 (4.0375, -21.4478) -> (7.0338, -22.4994)
  line L29 (7.0338, -22.4994) -> (7.6213, -25.62)
  line L30 (7.6213, -25.62) -> (5.2125, -27.6891)
  line L31 (5.2125, -27.6891) -> (2.2162, -26.6375)
  line L32 (2.2162, -26.6375) -> (1.6287, -23.5169)
  line L33 (-11.5002, -20.5778) -> (-8.3519, -20.1633)
  line L34 (-8.3519, -20.1633) -> (-6.4188, -22.6825)
  line L35 (-6.4188, -22.6825) -> (-7.634, -25.6162)
  line L36 (-7.634, -25.6162) -> (-10.7823, -26.0307)
  line L37 (-10.7823, -26.0307) -> (-12.7153, -23.5115)
  line L38 (-12.7153, -23.5115) -> (-11.5002, -20.5778)
  line L39 (-25.6162, -7.634) -> (-22.6825, -6.4188)
  line L40 (-22.6825, -6.4188) -> (-20.1633, -8.3519)
  line L41 (-20.1633, -8.3519) -> (-20.5778, -11.5002)
  line L42 (-20.5778, -11.5002) -> (-23.5115, -12.7153)
  line L43 (-23.5115, -12.7153) -> (-26.0307, -10.7823)
  line L44 (-26.0307, -10.7823) -> (-25.6162, -7.634)
  line L45 (22.6825, -6.4188) -> (20.5778, -11.5002)
  line L46 (20.5778, -11.5002) -> (7.3128, -6.0056)
  line L47 (7.3128, -6.0056) -> (9.4175, -0.9243)
  line L48 (9.4175, -0.9243) -> (22.6825, -6.4188)
  line L49 (7.0338, -22.4994) -> (1.6287, -23.5169)
  line L50 (1.6287, -23.5169) -> (-1.0275, -9.4068)
  line L51 (-1.0275, -9.4068) -> (4.3776, -8.3893)
  line L52 (4.3776, -8.3893) -> (7.0338, -22.4994)
  line L53 (-6.4188, -22.6825) -> (-11.5002, -20.5778)
  line L54 (-11.5002, -20.5778) -> (-6.0056, -7.3128)
  line L55 (-6.0056, -7.3128) -> (-0.9243, -9.4175)
  line L56 (-0.9243, -9.4175) -> (-6.4188, -22.6825)
  line L57 (-20.5778, -11.5002) -> (-22.6825, -6.4188)
  line L58 (-22.6825, -6.4188) -> (-9.4175, -0.9243)
  line L59 (-9.4175, -0.9243) -> (-7.3128, -6.0056)
  line L60 (-7.3128, -6.0056) -> (-20.5778, -11.5002)
  point P0 (0, 0)
  dimension "d153" = 5.5
  constraints: 110 end point, 11 parallel, 8 equal length, 6 coincident, 6 perpendicular, 6 point on line, 65 other
  measures "d153" distance between parallel lines of L8 L11
extrude "Extrusion18" cut sketch "Skizze33" against normal blind 3 contours A1 | A2 | A4 | A5 | A8 | L58 L59 L60 A12 | A12 L60 L41 L40 L58 | L48 L23 L22 L46 A12 | A12 L46 L47 L48 | L57 L42 L43 L44 L39 | L40 L41 L57 | L45 L22 L23 | L24 L25 L26 L21 L45 | L54 L55 L51 L50 L56 A12 | A12 L56 L34 L33 L54 | L14 L8 L7 L16 A12 | A12 L16 L52 L51 L15 L14 | L53 L35 L36 L37 L38 | L33 L34 L53 | L13 L7 L8 | L9 L10 L11 L6 L13 | L51 L52 L16 L15 | L15 L16 L52 A12 L50 L56 L55 L51 | A12 L52 L28 L27 L50 | L50 L51 L55 L56 | L49 L29 L30 L31 L32 | L27 L28 L49
mirror "Spiegeln4" about plane through (50, 0, 0) normal (0, 1, 0) of "Extrusion18"
